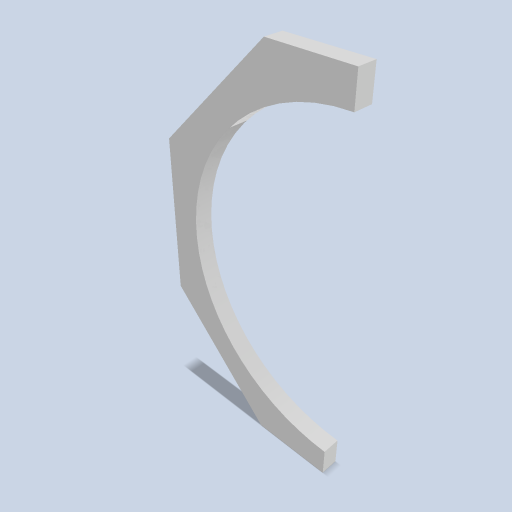
# Autodesk Inventor part: Tube Ring Half
Saved by Autodesk Inventor 2023 (Build 270158000, 158)
## iProperties
Created: 2022-10-10
Part Number: Tube Ring Half
Material: Generic
Document SubType Name: Modeling
Designer: Nathan
Density: 1 g/cm^3
Appearance: Default
Mass: 625.034 g
Surface Area: 1110.33 cm^2
Volume: 625.034 cm^3
Author: Nathan
Autodesk Inventor part; units mm, degrees
ref_plane "YZ Plane" through (0, 0, 0) normal (1, 0, 0) x (0, 1, 0)
ref_plane "XZ Plane" through (0, 0, 0) normal (0, 1, 0) x (-1, 0, 0)
ref_plane "XY Plane" through (0, 0, 0) normal (0, 0, 1) x (1, 0, 0)
sketch "Sketch1" plane through (0, 0, 0) normal (0, 0, 1) x (1, 0, 0)
  circle A0 centre (190.5, 190.5) radius 161.29
  circle A1 centre (190.5, 190.5) radius 161.29
  line L0 (0, 269.4113) -> (111.5887, 381)
  line L1 (0, 269.4113) -> (157.8102, 269.4113) construction
  line L2 (0, 111.5878) -> (111.5895, 0)
  line L3 (269.4113, 0) -> (381, 111.5903)
  line L4 (380.9968, 269.4113) -> (269.4113, 381)
  line L5 (0, 0) -> (380.9968, 0)
  line L6 (380.9968, 0) -> (380.9968, 380.9968)
  line L7 (380.9968, 380.9968) -> (0, 380.9968)
  line L8 (0, 380.9968) -> (0, 0)
  line L9 (190.4984, 380.9968) -> (190.4984, 351.79)
  line L10 (190.4984, 29.21) -> (190.4984, 0)
  point P0 (111.5855, 380.9968)
  point P1 (111.5895, 0)
  point P2 (380.9968, 111.5871)
  point P3 (269.4145, 380.9968)
  dimension "d3" = 322.58
  dimension "d27" = 45
  dimension "d28" = 157.8102
  dimension "d30" = 157.8235
  dimension "d32" = 157.8218
  dimension "d40" = 157.808
  dimension "d42" = 380.9968
  dimension "d43" = 380.9968
  dimension "d44" = 190.5
  dimension "d45" = 190.5
  dimension "d46" = 111.5878
  dimension "d49" = 29.21
  dimension "d50" = 29.2068
  dimension "d51" = 269.4113
  dimension "d52" = 381
  dimension "d53" = 269.4113
  dimension "d54" = 157.821
  dimension "d55" = 111.5887
  dimension "d56" = 269.4113
  dimension "d57" = 111.5878
  dimension "d58" = 111.5895
  dimension "d59" = 111.5855
  constraints: 22 end point, 2 centre point, 2 horizontal, 2 midpoint, 2 parallel, 2 perpendicular, 2 point on circle, 1 coincident, 1 concentric, 1 equal length, 1 point on line, 1 vertical
  measures "d3" diameter of A0
  measures "d27" angle of L1 L0
  measures "d28" distance of L0.start L0.end
  measures "d30" distance of L2.start L0.start
  measures "d32" distance of L3.start L2.end
  measures "d40" distance of L4.start L4.end
  measures "d42" distance of L6.end L7.end
  measures "d43" distance of L5.end L6.end
  measures "d44" horizontal distance of L5.start A1.centre
  measures "d45" horizontal distance of L5.start A0.centre
  measures "d46" vertical distance of L2.start L2.end
  measures "d49" distance of L10.start L10.end
  measures "d50" distance of L9.start L9.end
  measures "d51" distance from line of L5 L4.start
  measures "d52" vertical distance of L5.start L4.end
  measures "d53" distance of L7.end L4.end
  measures "d54" distance of L3.end L4.start
  measures "d55" distance of L7.end L0.end
  measures "d56" distance of L5.start L0.start
  measures "d57" distance from line of L5 L2.start
  measures "d58" distance of L5.start L2.end
  measures "d59" distance of L5.end L3.start
extrude "Extrusion3" add sketch "Sketch1" along normal blind 18.0086 contours A0 L10 L5 L2 L8 L0 L7 L9
body "Solid3"
